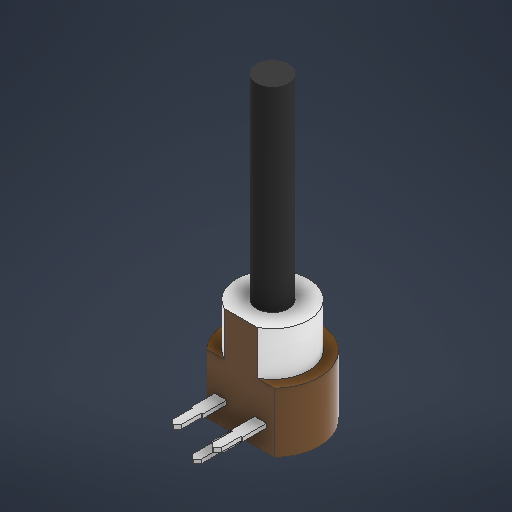
# Autodesk Inventor part: SMC10H04
Saved by Autodesk Inventor 2026 (Build 300175050, 175E)
## iProperties
Created: 2025-07-31
Part Number: SMC10H04
Material: Generic
Document SubType Name: Modeling
Designer: user
Density: 1 g/cm^3
Appearance: Default
Author: user
Autodesk Inventor part; units mm, degrees
ref_plane "YZ Plane" through (0, 0, 0) normal (1, 0, 0) x (0, 1, 0)
ref_plane "XZ Plane" through (0, 0, 0) normal (0, 1, 0) x (-1, 0, 0)
ref_plane "XY Plane" through (0, 0, 0) normal (0, 0, 1) x (1, 0, 0)
sketch "Sketch1" plane through (0, 0, 0) normal (0, 1, 0) x (-1, 0, 0)
  circle A0 centre (0, 0) radius 5.85
  line L0 (5, 0) -> (-5, 0)
  line L1 (-5, 0) -> (-5, 4)
  line L2 (-5, 4) -> (5, 4)
  line L3 (5, 4) -> (5, 0)
  point P0 (4.2688, 4)
  point P1 (-4.2688, 4)
  dimension "d0" = 11.7
  dimension "d1" = 4
  dimension "d2" = 10
  constraints: 8 end point, 3 coincident, 2 parallel, 1 centre point, 1 horizontal, 1 midpoint, 1 perpendicular
  measures "d0" diameter of A0
  measures "d1" distance from line of point (0, 0) L2
  measures "d2" distance of L1.end L2.end
extrude "Extrusion1" add sketch "Sketch1" along normal blind 7.5 contours A0 L1 L0 L3 | L3 L0 L1 A0 L2
sketch "Sketch2" plane through (0, 7.5, 0) normal (0, 1, 0) x (1, 0, 0)
  arc A0 (4.2688, -4) -> (-4.2688, -4) centre (0, 0) ccw projected
  circle A1 centre (0, 0) radius 4.5
  line L0 (-4.2688, -4) -> (4.2688, -4) projected
  arc A2 (4.2688, -4) -> (-4.2688, -4) centre (0, 0) ccw projected
  point P0 (-2.0616, -4)
  point P1 (2.0616, -4)
  dimension "d5" = 9
  constraints: 1 centre point, 1 coincident
  measures "d5" diameter of A1
extrude "Extrusion2" add sketch "Sketch2" along normal blind 5.5 contours L0 A1 picked at (-0.2884, 2.0732)
sketch "Sketch3" plane through (0, 13, 0) normal (0, 1, 0) x (1, 0, 0)
  circle A0 centre (0, 0) radius 2
  dimension "d8" = 4
  constraints: 1 centre point, 1 coincident
  measures "d8" diameter of A0
extrude "Extrusion3" add sketch "Sketch3" along normal blind 24.5
sketch "Sketch4" plane through (-4.2688, 0, 4) normal (0, 0, 1) x (1, 0, 0)
  line L0 (3.5188, 0.7) -> (5.0188, 0.7)
  line L1 (5.0188, 0.7) -> (5.0188, 0.2)
  line L2 (5.0188, 0.2) -> (3.5188, 0.2)
  line L3 (3.5188, 0.2) -> (3.5188, 0.7)
  line L4 (0, 0) -> (8.5376, 0) projected
  line L5 (6.3303, 7.5) -> (8.5376, 7.5) projected
  line L6 (1.0188, 3.2) -> (2.5188, 3.2)
  line L7 (2.5188, 3.2) -> (2.5188, 2.7)
  line L8 (2.5188, 2.7) -> (1.0188, 2.7)
  line L9 (1.0188, 2.7) -> (1.0188, 3.2)
  line L10 (6.0188, 3.2) -> (7.5188, 3.2)
  line L11 (7.5188, 3.2) -> (7.5188, 2.7)
  line L12 (7.5188, 2.7) -> (6.0188, 2.7)
  line L13 (6.0188, 2.7) -> (6.0188, 3.2)
  point P0 (4.2688, 0)
  point P1 (4.2688, 0)
  point P2 (4.2688, 0.2)
  point P3 (5.0188, 0.45)
  point P4 (2.5188, 2.95)
  point P5 (6.0188, 2.95)
  point P6 (3.5188, 0.45)
  point P7 (1.0188, 2.95)
  point P8 (6.7688, 2.7)
  point P9 (1.7688, 2.7)
  dimension "d11" = 0.5
  dimension "d12" = 1.5
  dimension "d13" = 7.05
  dimension "d14" = 2.5
  dimension "d15" = 2.5
  dimension "d16" = 2.5
  constraints: 24 end point, 10 parallel, 9 midpoint, 3 horizontal, 3 perpendicular, 1 horizontal alignment, 1 vertical alignment
  measures "d11" distance of L2.end L0.start
  measures "d12" distance of L1.end L2.end
  measures "d13" distance from line of L5 point (5.019, 0.45)
  measures "d14" horizontal distance of point (3.519, 0.45) point (1.019, 2.95)
  measures "d15" horizontal distance of point (6.769, 2.7) point (4.269, 0.2)
  measures "d16" horizontal distance of point (4.269, 0.2) point (1.769, 2.7)
extrude "Extrusion4" add sketch "Sketch4" along normal blind 3
sketch "Sketch5" plane through (-4.2688, 0, 7) normal (0, 0, 1) x (1, 0, 0)
  line L0 (1.0188, 3.2) -> (2.5188, 3.2) projected
  line L1 (1.2188, 3.2) -> (2.3188, 3.2)
  line L2 (2.3188, 3.2) -> (2.3188, 2.7)
  line L3 (2.3188, 2.7) -> (1.2188, 2.7)
  line L4 (1.2188, 2.7) -> (1.2188, 3.2)
  line L5 (1.0188, 2.7) -> (2.5188, 2.7) projected
  line L6 (7.5188, 3.2) -> (6.0188, 3.2) projected
  line L7 (6.2188, 3.2) -> (7.3188, 3.2)
  line L8 (7.3188, 3.2) -> (7.3188, 2.7)
  line L9 (7.3188, 2.7) -> (6.2188, 2.7)
  line L10 (6.2188, 2.7) -> (6.2188, 3.2)
  line L11 (3.5188, 0.7) -> (5.0188, 0.7) projected
  line L12 (3.7188, 0.7) -> (4.8188, 0.7)
  line L13 (4.8188, 0.7) -> (4.8188, 0.2)
  line L14 (4.8188, 0.2) -> (3.7188, 0.2)
  line L15 (3.7188, 0.2) -> (3.7188, 0.7)
  line L16 (6.0188, 2.7) -> (7.5188, 2.7) projected
  line L17 (3.5188, 0.2) -> (5.0188, 0.2) projected
  point P0 (4.2688, 0)
  point P1 (1.7688, 2.7)
  point P2 (2.3188, 2.95)
  point P3 (6.7688, 2.7)
  point P4 (4.2688, 0.2)
  point P5 (7.3188, 2.95)
  point P6 (6.2188, 2.95)
  dimension "d19" = 1.1
  dimension "d20" = 1.1
  dimension "d21" = 1.1
  constraints: 24 end point, 9 midpoint, 6 parallel, 3 horizontal, 3 perpendicular, 3 point on line
  measures "d19" distance from line of point (2.319, 2.95) L4
  measures "d20" distance of point (7.319, 2.95) point (6.219, 2.95)
  measures "d21" distance between parallel lines of L13 L15
extrude "Extrusion5" add sketch "Sketch5" along normal blind 3
chamfer "Chamfer1" distance 0.5 angle 45 6 edges at (-3.05, 2.95, 10) (-1.95, 2.95, 10) (-0.55, 0.45, 10) (0.55, 0.45, 10) (1.95, 2.95, 10) (3.05, 2.95, 10)
body "Solid1"
